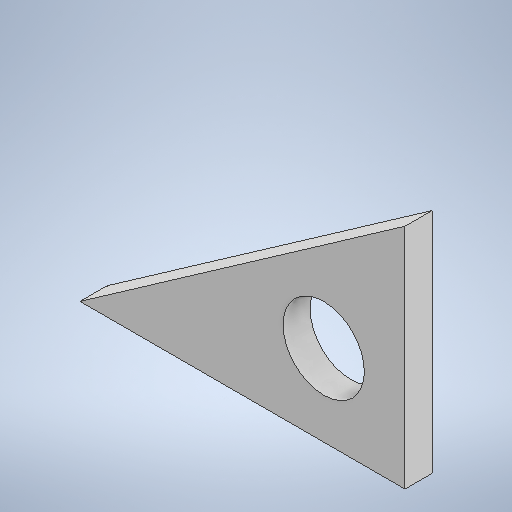
# Autodesk Inventor part: triangle
Saved by Autodesk Inventor 2025.1 (Build 291241000, 241)
## iProperties
Created: 2024-11-06
Part Number: triangle
Material: Generic
Document SubType Name: Modeling
Designer: bless
Density: 1 g/cm^3
Appearance: Default
Author: bless
Autodesk Inventor part; units mm, degrees
ref_plane "YZ Plane" through (0, 0, 0) normal (1, 0, 0) x (0, 1, 0)
ref_plane "XZ Plane" through (0, 0, 0) normal (0, 1, 0) x (-1, 0, 0)
ref_plane "XY Plane" through (0, 0, 0) normal (0, 0, 1) x (1, 0, 0)
sketch "Sketch1" plane through (0, 0, 0) normal (0, 0, 1) x (1, 0, 0)
  line L0 (-45.7835, -10.1388) -> (30.4165, -10.1388)
  line L1 (30.4165, -10.1388) -> (30.4165, 43.217)
  line L2 (30.4165, 43.217) -> (-45.7835, -10.1388)
  circle A0 centre (11.3665, 8.9112) radius 9.525
  point P0 (0, 0)
  dimension "d0" = 76.2
  dimension "d1" = 35
  dimension "d2" = 19.05
  dimension "d3" = 19.05
  dimension "d4" = 19.05
  constraints: 6 end point, 1 centre point, 1 horizontal, 1 vertical, 1 other
  measures "d0" distance of L0.start L0.end
  measures "d1" angle of L2 L0
  measures "d2" diameter of A0
  measures "d3" distance from line of L0 A0.centre
  measures "d4" distance from line of L1 A0.centre
extrude "Extrusion1" add sketch "Sketch1" along normal blind 6.35
body "Solid1"
